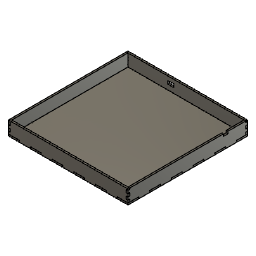
Laser cut Electronic box case v5 (Autodesk Fusion 360 design; units mm, degrees)
Autodesk Fusion 360 part; units mm, degrees
box "BoxPrimitive1" add length 215 width 215 height 3 placed x (0, 0, -1) y (-1, 0, 0) z (0, 1, 0) at (215, 0, 0) makes body 1
sketch "Sketch2" plane through (0, 0, 0) normal (0, 0, 1) x (1, 0, 0)
  line L0 (0, 3) -> (0, 0)
  line L1 (0, 0) -> (215, 0)
  line L2 (215, 0) -> (215, 3)
  line L3 (215, 3) -> (0, 3)
  line L4 (19.5455, 0) -> (39.0909, 0)
  line L5 (39.0909, 0) -> (39.0909, 3)
  line L6 (39.0909, 3) -> (19.5455, 3)
  line L7 (19.5455, 3) -> (19.5455, 0)
  dimension "d19" = 19.5455
  dimension "d20" = 3
  dimension "d21" = 19.5455
  constraint horizontal L4
  constraint vertical L5
  constraint horizontal L6
  constraint vertical L7
  constraint coincident L1 L4.start
  measures "d19" distance of L4.start L4.end
  measures "d20" distance of L4.start L6.end
  measures "d21" distance of L0.start L6.end
extrude "Extrude1" cut sketch "Sketch2" against normal blind 3 contours L1 L3 L4 L5 L6 L7 bodies 1
pattern_linear "R-Pattern1" count 5 spacing 39.0909 along (1, 0, 0) of 3 faces at (19.5455, 1, -2) (26.0606, 2, -3) (39.0909, 2, -2) on bodies 1
sketch "Sketch3" plane through (0, 0, 0) normal (-1, 0, 0) x (0, 0, 1)
  line L0 (-215, 3) -> (-215, 0)
  line L1 (-215, 0) -> (0, 0)
  line L2 (0, 0) -> (0, 3)
  line L3 (0, 3) -> (-215, 3)
  line L4 (-19.5455, 0) -> (-39.0909, 0)
  line L5 (-39.0909, 0) -> (-39.0909, 3)
  line L6 (-39.0909, 3) -> (-19.5455, 3)
  line L7 (-19.5455, 3) -> (-19.5455, 0)
  dimension "d28" = 19.5455
  dimension "d29" = 3
  dimension "d30" = 19.5455
  constraint horizontal L4
  constraint vertical L5
  constraint horizontal L6
  constraint vertical L7
  constraint coincident L1 L4.start
  measures "d28" distance of L4.start L4.end
  measures "d29" distance of L4.start L6.end
  measures "d30" distance of L2.end L6.end
extrude "Extrude2" cut sketch "Sketch3" against normal blind 3 contours L1 L3 L4 L5 L6 L7 bodies 1
pattern_linear "R-Pattern2" count 5 spacing 39.0909 along (0, 0, -1) of 3 faces at (2, 2, -39.0909) (3, 2, -32.5758) (2, 1, -19.5455) on bodies 1
sketch "Sketch4" plane through (0, 0, 0) normal (0, 0, 1) x (1, 0, 0)
  line L0 (0, 0) -> (215, 0)
  line L1 (215, 0) -> (215, 25)
  line L2 (215, 25) -> (0, 25)
  line L3 (0, 25) -> (0, 0)
  dimension "d37" = 215
  dimension "d38" = 25
  constraint horizontal L0
  constraint vertical L1
  constraint horizontal L2
  constraint vertical L3
  constraint coincident L0.start L3.end
  measures "d37" distance of L0.start L0.end
  measures "d38" distance of L0.start L2.end
extrude "Extrude3" add sketch "Sketch4" against normal blind 3 separate body makes body 2
combine "Combine1" operation cut target body 2 tool bodies 1 keep tools
sketch "Sketch6" plane through (0, 0, 0) normal (-1, 0, 0) x (0, 0, 1)
  line L0 (-3, 3) -> (0, 3)
  line L1 (0, 3) -> (0, 25)
  line L2 (0, 25) -> (-3, 25)
  line L3 (-3, 25) -> (-3, 3)
  line L4 (-3, 7.6) -> (0, 7.6)
  line L5 (0, 7.6) -> (0, 12.6)
  line L6 (0, 12.6) -> (-3, 12.6)
  line L7 (-3, 12.6) -> (-3, 7.6)
  dimension "d52" = 3
  dimension "d53" = 5
  constraint horizontal L4
  constraint vertical L5
  constraint horizontal L6
  constraint vertical L7
  constraint coincident L3 L4.start
  measures "d52" distance of L4.start L4.end
  measures "d53" distance of L4.start L6.end
extrude "Extrude7" cut sketch "Sketch6" against normal blind 3 contours L1 L3 L4 L5 L6 L7 bodies 2
pattern_linear "R-Pattern3" count 2 spacing 10 along (0, 1, 0) of 3 faces at (2, 7.6, -1) (3, 10.9333, -2) (2, 12.6, -2) on bodies 2
extrude "Extrude8" add 1 faces at (97.7273, 17.6667, -3) along direction (0, 0, 1) blind 3 from surface at -212 separate body on bodies 2 makes body 3
combine "Combine5" operation cut target body 1 tool bodies 3 keep tools
sketch "Sketch7" plane through (0, 0, 0) normal (1, 0, 0) x (0, 0, -1)
  line L0 (0, 0) -> (215, 0)
  line L1 (215, 0) -> (215, 25)
  line L2 (215, 25) -> (0, 25)
  line L3 (0, 25) -> (0, 0)
  dimension "d63" = 215
  dimension "d64" = 25
  constraint horizontal L0
  constraint vertical L1
  constraint horizontal L2
  constraint vertical L3
  constraint coincident L0.start L3.end
  measures "d63" distance of L0.start L0.end
  measures "d64" distance of L0.start L2.end
extrude "Extrude9" add sketch "Sketch7" along normal blind 3 separate body makes body 4
combine "Combine6" operation cut target body 4 tool bodies 3 1 2 keep tools
extrude "Extrude10" add 1 faces at (3, 17.6667, -97.7273) along direction (-1, 0, 0) blind 3 from surface at -212 separate body on bodies 4 makes body 5
combine "Combine7" operation cut target body 1 tool bodies 5 keep tools
combine "Combine8" operation cut target body 3 tool bodies 5 keep tools
combine "Combine9" operation cut target body 2 tool bodies 5 keep tools
sketch "Sketch8" plane through (215, 0, 0) normal (1, 0, 0) x (0, 0, -1)
  line L0 (212, 25) -> (3, 25)
  line L1 (3, 25) -> (3, 22.6)
  line L2 (3, 22.6) -> (0, 22.6)
  line L3 (0, 22.6) -> (0, 17.6)
  line L4 (0, 17.6) -> (3, 17.6)
  line L5 (3, 17.6) -> (3, 12.6)
  line L6 (3, 12.6) -> (0, 12.6)
  line L7 (0, 12.6) -> (0, 7.6)
  line L8 (0, 7.6) -> (3, 7.6)
  line L9 (3, 7.6) -> (3, 3)
  line L10 (3, 3) -> (19.5455, 3)
  line L11 (19.5455, 3) -> (19.5455, 0)
  line L12 (19.5455, 0) -> (39.0909, 0)
  line L13 (39.0909, 0) -> (39.0909, 3)
  line L14 (39.0909, 3) -> (58.6364, 3)
  line L15 (58.6364, 3) -> (58.6364, 0)
  line L16 (58.6364, 0) -> (78.1818, 0)
  line L17 (78.1818, 0) -> (78.1818, 3)
  line L18 (78.1818, 3) -> (97.7273, 3)
  line L19 (97.7273, 3) -> (97.7273, 0)
  line L20 (97.7273, 0) -> (117.2727, 0)
  line L21 (117.2727, 0) -> (117.2727, 3)
  line L22 (117.2727, 3) -> (136.8182, 3)
  line L23 (136.8182, 3) -> (136.8182, 0)
  line L24 (136.8182, 0) -> (156.3636, 0)
  line L25 (156.3636, 0) -> (156.3636, 3)
  line L26 (156.3636, 3) -> (175.9091, 3)
  line L27 (175.9091, 3) -> (175.9091, 0)
  line L28 (175.9091, 0) -> (195.4545, 0)
  line L29 (195.4545, 0) -> (195.4545, 3)
  line L30 (195.4545, 3) -> (212, 3)
  line L31 (212, 3) -> (212, 7.6)
  line L32 (212, 7.6) -> (215, 7.6)
  line L33 (215, 12.6) -> (212, 12.6)
  line L34 (212, 12.6) -> (212, 17.6)
  line L35 (212, 17.6) -> (215, 17.6)
  line L36 (215, 17.6) -> (215, 22.6)
  line L37 (215, 22.6) -> (212, 22.6)
  line L38 (212, 22.6) -> (212, 25)
  line L39 (179.8983, 25) -> (171.8983, 25)
  line L40 (171.8983, 25) -> (171.8983, 21)
  line L41 (171.8983, 21) -> (179.8983, 21)
  line L42 (179.8983, 21) -> (179.8983, 25)
  line L43 (215, 7.6) -> (215, 12.6)
  dimension "d72" = 8
  dimension "d73" = 4
  constraint horizontal L39
  constraint vertical L40
  constraint horizontal L41
  constraint vertical L42
  constraint coincident L0 L39.start
  measures "d72" distance of L39.start L39.end
  measures "d73" distance of L39.start L41.end
extrude "Extrude11" cut sketch "Sketch8" against normal blind 3 contours L0 L39 L40 L41 L42 bodies 5
sketch "Sketch9" plane through (0, 0, -215) normal (0, 0, -1) x (-1, 0, 0)
  line L0 (-212, 7.6) -> (-215, 7.6)
  line L1 (-215, 7.6) -> (-215, 3)
  line L2 (-215, 3) -> (-195.4545, 3)
  line L3 (-195.4545, 3) -> (-195.4545, 0)
  line L4 (-195.4545, 0) -> (-175.9091, 0)
  line L5 (-175.9091, 0) -> (-175.9091, 3)
  line L6 (-175.9091, 3) -> (-156.3636, 3)
  line L7 (-156.3636, 3) -> (-156.3636, 0)
  line L8 (-156.3636, 0) -> (-136.8182, 0)
  line L9 (-136.8182, 0) -> (-136.8182, 3)
  line L10 (-136.8182, 3) -> (-117.2727, 3)
  line L11 (-117.2727, 3) -> (-117.2727, 0)
  line L12 (-117.2727, 0) -> (-97.7273, 0)
  line L13 (-97.7273, 0) -> (-97.7273, 3)
  line L14 (-97.7273, 3) -> (-78.1818, 3)
  line L15 (-78.1818, 3) -> (-78.1818, 0)
  line L16 (-78.1818, 0) -> (-58.6364, 0)
  line L17 (-58.6364, 0) -> (-58.6364, 3)
  line L18 (-58.6364, 3) -> (-39.0909, 3)
  line L19 (-39.0909, 3) -> (-39.0909, 0)
  line L20 (-39.0909, 0) -> (-19.5455, 0)
  line L21 (-19.5455, 0) -> (-19.5455, 3)
  line L22 (-19.5455, 3) -> (0, 3)
  line L23 (0, 3) -> (0, 7.6)
  line L24 (0, 7.6) -> (-3, 7.6)
  line L25 (-3, 7.6) -> (-3, 12.6)
  line L26 (-3, 12.6) -> (0, 12.6)
  line L27 (0, 12.6) -> (0, 17.6)
  line L28 (0, 17.6) -> (-3, 17.6)
  line L29 (-3, 17.6) -> (-3, 22.6)
  line L30 (-3, 22.6) -> (0, 22.6)
  line L31 (0, 22.6) -> (0, 25)
  line L32 (0, 25) -> (-215, 25)
  line L33 (-215, 22.6) -> (-212, 22.6)
  line L34 (-212, 22.6) -> (-212, 17.6)
  line L35 (-212, 17.6) -> (-215, 17.6)
  line L36 (-215, 12.6) -> (-212, 12.6)
  line L37 (-74.7061, 17.8863) -> (-85.2061, 17.8863)
  line L38 (-85.2061, 17.8863) -> (-85.2061, 12.1863)
  line L39 (-85.2061, 12.1863) -> (-74.7061, 12.1863)
  line L40 (-74.7061, 12.1863) -> (-74.7061, 17.8863)
  line L41 (-74.7061, 17.8863) -> (-85.2061, 12.1863) construction
  line L42 (-85.2061, 17.8863) -> (-74.7061, 12.1863) construction
  line L43 (-215, 25) -> (-215, 22.6)
  line L44 (-215, 17.6) -> (-215, 12.6)
  line L45 (-212, 12.6) -> (-212, 7.6)
  point P0 (-79.9561, 15.0363)
  dimension "d78" = 10.5
  dimension "d79" = 5.7
  constraint horizontal L37
  constraint perpendicular L37 L38
  constraint parallel L37 L39
  constraint parallel L38 L40
  constraint coincident L41 P0
  constraint coincident L42 P0
  measures "d78" distance of L38.end L39.end
  measures "d79" distance of L37.end L38.end
extrude "Extrude12" cut sketch "Sketch9" against normal blind 3 contours L37 L38 L39 L40 bodies 3
sketch "Base DXF" plane through (0, 3, 0) normal (0, 1, 0) x (-1, 0, 0)
  line L0 (-215, 0) -> (-215, -19.5455)
  line L1 (-215, -19.5455) -> (-212, -19.5455)
  line L2 (-212, -19.5455) -> (-212, -39.0909)
  line L3 (-212, -39.0909) -> (-215, -39.0909)
  line L4 (-215, -39.0909) -> (-215, -58.6364)
  line L5 (-215, -58.6364) -> (-212, -58.6364)
  line L6 (-212, -58.6364) -> (-212, -78.1818)
  line L7 (-212, -78.1818) -> (-215, -78.1818)
  line L8 (-215, -78.1818) -> (-215, -97.7273)
  line L9 (-215, -97.7273) -> (-212, -97.7273)
  line L10 (-212, -97.7273) -> (-212, -117.2727)
  line L11 (-212, -117.2727) -> (-215, -117.2727)
  line L12 (-215, -117.2727) -> (-215, -136.8182)
  line L13 (-215, -136.8182) -> (-212, -136.8182)
  line L14 (-212, -136.8182) -> (-212, -156.3636)
  line L15 (-212, -156.3636) -> (-215, -156.3636)
  line L16 (-215, -156.3636) -> (-215, -175.9091)
  line L17 (-215, -175.9091) -> (-212, -175.9091)
  line L18 (-212, -175.9091) -> (-212, -195.4545)
  line L19 (-212, -195.4545) -> (-215, -195.4545)
  line L20 (-215, -195.4545) -> (-215, -215)
  line L21 (-215, -215) -> (-195.4545, -215)
  line L22 (-195.4545, -215) -> (-195.4545, -212)
  line L23 (-195.4545, -212) -> (-175.9091, -212)
  line L24 (-175.9091, -212) -> (-175.9091, -215)
  line L25 (-175.9091, -215) -> (-156.3636, -215)
  line L26 (-156.3636, -215) -> (-156.3636, -212)
  line L27 (-156.3636, -212) -> (-136.8182, -212)
  line L28 (-136.8182, -212) -> (-136.8182, -215)
  line L29 (-136.8182, -215) -> (-117.2727, -215)
  line L30 (-117.2727, -215) -> (-117.2727, -212)
  line L31 (-117.2727, -212) -> (-97.7273, -212)
  line L32 (-97.7273, -212) -> (-97.7273, -215)
  line L33 (-97.7273, -215) -> (-78.1818, -215)
  line L34 (-78.1818, -215) -> (-78.1818, -212)
  line L35 (-78.1818, -212) -> (-58.6364, -212)
  line L36 (-58.6364, -212) -> (-58.6364, -215)
  line L37 (-58.6364, -215) -> (-39.0909, -215)
  line L38 (-39.0909, -215) -> (-39.0909, -212)
  line L39 (-39.0909, -212) -> (-19.5455, -212)
  line L40 (-19.5455, -212) -> (-19.5455, -215)
  line L41 (-19.5455, -215) -> (0, -215)
  line L42 (0, -215) -> (0, -195.4545)
  line L43 (0, -195.4545) -> (-3, -195.4545)
  line L44 (-3, -195.4545) -> (-3, -175.9091)
  line L45 (-3, -175.9091) -> (0, -175.9091)
  line L46 (0, -175.9091) -> (0, -156.3636)
  line L47 (0, -156.3636) -> (-3, -156.3636)
  line L48 (-3, -156.3636) -> (-3, -136.8182)
  line L49 (-3, -136.8182) -> (0, -136.8182)
  line L50 (0, -136.8182) -> (0, -117.2727)
  line L51 (0, -117.2727) -> (-3, -117.2727)
  line L52 (-3, -117.2727) -> (-3, -97.7273)
  line L53 (-3, -97.7273) -> (0, -97.7273)
  line L54 (0, -97.7273) -> (0, -78.1818)
  line L55 (0, -78.1818) -> (-3, -78.1818)
  line L56 (-3, -78.1818) -> (-3, -58.6364)
  line L57 (-3, -58.6364) -> (0, -58.6364)
  line L58 (0, -58.6364) -> (0, -39.0909)
  line L59 (0, -39.0909) -> (-3, -39.0909)
  line L60 (-3, -39.0909) -> (-3, -19.5455)
  line L61 (-3, -19.5455) -> (0, -19.5455)
  line L62 (0, -19.5455) -> (0, 0)
  line L63 (0, 0) -> (-19.5455, 0)
  line L64 (-19.5455, 0) -> (-19.5455, -3)
  line L65 (-19.5455, -3) -> (-39.0909, -3)
  line L66 (-39.0909, -3) -> (-39.0909, 0)
  line L67 (-39.0909, 0) -> (-58.6364, 0)
  line L68 (-58.6364, 0) -> (-58.6364, -3)
  line L69 (-58.6364, -3) -> (-78.1818, -3)
  line L70 (-78.1818, -3) -> (-78.1818, 0)
  line L71 (-78.1818, 0) -> (-97.7273, 0)
  line L72 (-97.7273, 0) -> (-97.7273, -3)
  line L73 (-97.7273, -3) -> (-117.2727, -3)
  line L74 (-117.2727, -3) -> (-117.2727, 0)
  line L75 (-117.2727, 0) -> (-136.8182, 0)
  line L76 (-136.8182, 0) -> (-136.8182, -3)
  line L77 (-136.8182, -3) -> (-156.3636, -3)
  line L78 (-156.3636, -3) -> (-156.3636, 0)
  line L79 (-156.3636, 0) -> (-175.9091, 0)
  line L80 (-175.9091, 0) -> (-175.9091, -3)
  line L81 (-175.9091, -3) -> (-195.4545, -3)
  line L82 (-195.4545, -3) -> (-195.4545, 0)
  line L83 (-195.4545, 0) -> (-215, 0)
sketch "Front DXF" plane through (0, 0, 0) normal (0, 0, 1) x (1, 0, 0)
  line L0 (212, 22.6) -> (215, 22.6)
  line L1 (215, 22.6) -> (215, 25)
  line L2 (215, 25) -> (0, 25)
  line L3 (0, 25) -> (0, 22.6)
  line L4 (0, 22.6) -> (3, 22.6)
  line L5 (3, 22.6) -> (3, 17.6)
  line L6 (3, 17.6) -> (0, 17.6)
  line L7 (0, 17.6) -> (0, 12.6)
  line L8 (0, 12.6) -> (3, 12.6)
  line L9 (3, 12.6) -> (3, 7.6)
  line L10 (3, 7.6) -> (0, 7.6)
  line L11 (0, 7.6) -> (0, 3)
  line L12 (0, 3) -> (19.5455, 3)
  line L13 (19.5455, 3) -> (19.5455, 0)
  line L14 (19.5455, 0) -> (39.0909, 0)
  line L15 (39.0909, 0) -> (39.0909, 3)
  line L16 (39.0909, 3) -> (58.6364, 3)
  line L17 (58.6364, 3) -> (58.6364, 0)
  line L18 (58.6364, 0) -> (78.1818, 0)
  line L19 (78.1818, 0) -> (78.1818, 3)
  line L20 (78.1818, 3) -> (97.7273, 3)
  line L21 (97.7273, 3) -> (97.7273, 0)
  line L22 (97.7273, 0) -> (117.2727, 0)
  line L23 (117.2727, 0) -> (117.2727, 3)
  line L24 (117.2727, 3) -> (136.8182, 3)
  line L25 (136.8182, 3) -> (136.8182, 0)
  line L26 (136.8182, 0) -> (156.3636, 0)
  line L27 (156.3636, 0) -> (156.3636, 3)
  line L28 (156.3636, 3) -> (175.9091, 3)
  line L29 (175.9091, 3) -> (175.9091, 0)
  line L30 (175.9091, 0) -> (195.4545, 0)
  line L31 (195.4545, 0) -> (195.4545, 3)
  line L32 (195.4545, 3) -> (215, 3)
  line L33 (215, 3) -> (215, 7.6)
  line L34 (215, 7.6) -> (212, 7.6)
  line L35 (212, 7.6) -> (212, 12.6)
  line L36 (212, 12.6) -> (215, 12.6)
  line L37 (215, 12.6) -> (215, 17.6)
  line L38 (215, 17.6) -> (212, 17.6)
  line L39 (212, 17.6) -> (212, 22.6)
sketch "Back DXF" plane through (0, 0, -215) normal (0, 0, -1) x (-1, 0, 0)
  line L0 (-85.2061, 17.8863) -> (-74.7061, 17.8863)
  line L1 (-74.7061, 17.8863) -> (-74.7061, 12.1863)
  line L2 (-74.7061, 12.1863) -> (-85.2061, 12.1863)
  line L3 (-85.2061, 12.1863) -> (-85.2061, 17.8863)
  line L4 (-212, 7.6) -> (-215, 7.6)
  line L5 (-215, 7.6) -> (-215, 3)
  line L6 (-215, 3) -> (-195.4545, 3)
  line L7 (-195.4545, 3) -> (-195.4545, 0)
  line L8 (-195.4545, 0) -> (-175.9091, 0)
  line L9 (-175.9091, 0) -> (-175.9091, 3)
  line L10 (-175.9091, 3) -> (-156.3636, 3)
  line L11 (-156.3636, 3) -> (-156.3636, 0)
  line L12 (-156.3636, 0) -> (-136.8182, 0)
  line L13 (-136.8182, 0) -> (-136.8182, 3)
  line L14 (-136.8182, 3) -> (-117.2727, 3)
  line L15 (-117.2727, 3) -> (-117.2727, 0)
  line L16 (-117.2727, 0) -> (-97.7273, 0)
  line L17 (-97.7273, 0) -> (-97.7273, 3)
  line L18 (-97.7273, 3) -> (-78.1818, 3)
  line L19 (-78.1818, 3) -> (-78.1818, 0)
  line L20 (-78.1818, 0) -> (-58.6364, 0)
  line L21 (-58.6364, 0) -> (-58.6364, 3)
  line L22 (-58.6364, 3) -> (-39.0909, 3)
  line L23 (-39.0909, 3) -> (-39.0909, 0)
  line L24 (-39.0909, 0) -> (-19.5455, 0)
  line L25 (-19.5455, 0) -> (-19.5455, 3)
  line L26 (-19.5455, 3) -> (0, 3)
  line L27 (0, 3) -> (0, 7.6)
  line L28 (0, 7.6) -> (-3, 7.6)
  line L29 (-3, 7.6) -> (-3, 12.6)
  line L30 (-3, 12.6) -> (0, 12.6)
  line L31 (0, 12.6) -> (0, 17.6)
  line L32 (0, 17.6) -> (-3, 17.6)
  line L33 (-3, 17.6) -> (-3, 22.6)
  line L34 (-3, 22.6) -> (0, 22.6)
  line L35 (0, 22.6) -> (0, 25)
  line L36 (0, 25) -> (-215, 25)
  line L37 (-215, 25) -> (-215, 22.6)
  line L38 (-215, 22.6) -> (-212, 22.6)
  line L39 (-212, 22.6) -> (-212, 17.6)
  line L40 (-212, 17.6) -> (-215, 17.6)
  line L41 (-215, 17.6) -> (-215, 12.6)
  line L42 (-215, 12.6) -> (-212, 12.6)
  line L43 (-212, 12.6) -> (-212, 7.6)
sketch "Right DXF" plane through (215, 0, 0) normal (1, 0, 0) x (0, 0, -1)
  line L0 (171.8983, 21) -> (171.8983, 25)
  line L1 (171.8983, 25) -> (3, 25)
  line L2 (3, 25) -> (3, 22.6)
  line L3 (3, 22.6) -> (0, 22.6)
  line L4 (0, 22.6) -> (0, 17.6)
  line L5 (0, 17.6) -> (3, 17.6)
  line L6 (3, 17.6) -> (3, 12.6)
  line L7 (3, 12.6) -> (0, 12.6)
  line L8 (0, 12.6) -> (0, 7.6)
  line L9 (0, 7.6) -> (3, 7.6)
  line L10 (3, 7.6) -> (3, 3)
  line L11 (3, 3) -> (19.5455, 3)
  line L12 (19.5455, 3) -> (19.5455, 0)
  line L13 (19.5455, 0) -> (39.0909, 0)
  line L14 (39.0909, 0) -> (39.0909, 3)
  line L15 (39.0909, 3) -> (58.6364, 3)
  line L16 (58.6364, 3) -> (58.6364, 0)
  line L17 (58.6364, 0) -> (78.1818, 0)
  line L18 (78.1818, 0) -> (78.1818, 3)
  line L19 (78.1818, 3) -> (97.7273, 3)
  line L20 (97.7273, 3) -> (97.7273, 0)
  line L21 (97.7273, 0) -> (117.2727, 0)
  line L22 (117.2727, 0) -> (117.2727, 3)
  line L23 (117.2727, 3) -> (136.8182, 3)
  line L24 (136.8182, 3) -> (136.8182, 0)
  line L25 (136.8182, 0) -> (156.3636, 0)
  line L26 (156.3636, 0) -> (156.3636, 3)
  line L27 (156.3636, 3) -> (175.9091, 3)
  line L28 (175.9091, 3) -> (175.9091, 0)
  line L29 (175.9091, 0) -> (195.4545, 0)
  line L30 (195.4545, 0) -> (195.4545, 3)
  line L31 (195.4545, 3) -> (212, 3)
  line L32 (212, 3) -> (212, 7.6)
  line L33 (212, 7.6) -> (215, 7.6)
  line L34 (215, 7.6) -> (215, 12.6)
  line L35 (215, 12.6) -> (212, 12.6)
  line L36 (212, 12.6) -> (212, 17.6)
  line L37 (212, 17.6) -> (215, 17.6)
  line L38 (215, 17.6) -> (215, 22.6)
  line L39 (215, 22.6) -> (212, 22.6)
  line L40 (212, 22.6) -> (212, 25)
  line L41 (212, 25) -> (179.8983, 25)
  line L42 (179.8983, 25) -> (179.8983, 21)
  line L43 (179.8983, 21) -> (171.8983, 21)
sketch "Left DXF" plane through (0, 0, 0) normal (-1, 0, 0) x (0, 0, 1)
  line L0 (-3, 22.6) -> (-3, 25)
  line L1 (-3, 25) -> (-212, 25)
  line L2 (-212, 25) -> (-212, 22.6)
  line L3 (-212, 22.6) -> (-215, 22.6)
  line L4 (-215, 22.6) -> (-215, 17.6)
  line L5 (-215, 17.6) -> (-212, 17.6)
  line L6 (-212, 17.6) -> (-212, 12.6)
  line L7 (-212, 12.6) -> (-215, 12.6)
  line L8 (-215, 12.6) -> (-215, 7.6)
  line L9 (-215, 7.6) -> (-212, 7.6)
  line L10 (-212, 7.6) -> (-212, 3)
  line L11 (-212, 3) -> (-195.4545, 3)
  line L12 (-195.4545, 3) -> (-195.4545, 0)
  line L13 (-195.4545, 0) -> (-175.9091, 0)
  line L14 (-175.9091, 0) -> (-175.9091, 3)
  line L15 (-175.9091, 3) -> (-156.3636, 3)
  line L16 (-156.3636, 3) -> (-156.3636, 0)
  line L17 (-156.3636, 0) -> (-136.8182, 0)
  line L18 (-136.8182, 0) -> (-136.8182, 3)
  line L19 (-136.8182, 3) -> (-117.2727, 3)
  line L20 (-117.2727, 3) -> (-117.2727, 0)
  line L21 (-117.2727, 0) -> (-97.7273, 0)
  line L22 (-97.7273, 0) -> (-97.7273, 3)
  line L23 (-97.7273, 3) -> (-78.1818, 3)
  line L24 (-78.1818, 3) -> (-78.1818, 0)
  line L25 (-78.1818, 0) -> (-58.6364, 0)
  line L26 (-58.6364, 0) -> (-58.6364, 3)
  line L27 (-58.6364, 3) -> (-39.0909, 3)
  line L28 (-39.0909, 3) -> (-39.0909, 0)
  line L29 (-39.0909, 0) -> (-19.5455, 0)
  line L30 (-19.5455, 0) -> (-19.5455, 3)
  line L31 (-19.5455, 3) -> (-3, 3)
  line L32 (-3, 3) -> (-3, 7.6)
  line L33 (-3, 7.6) -> (0, 7.6)
  line L34 (0, 7.6) -> (0, 12.6)
  line L35 (0, 12.6) -> (-3, 12.6)
  line L36 (-3, 12.6) -> (-3, 17.6)
  line L37 (-3, 17.6) -> (0, 17.6)
  line L38 (0, 17.6) -> (0, 22.6)
  line L39 (0, 22.6) -> (-3, 22.6)
equation "Length = 215 mm"
equation "Width = 215 mm"
equation "Height = 25 mm"
equation "Thickness = 3 mm"
equation "LSTab = 5"
equation "WSTab = 5"
equation "HSTab = 2"
equation "LTabForm = Length / ( ( LSTab * 2 ) + 1 )"
equation "WTabForm = Width / ( ( WSTab * 2 ) + 1 )"
equation "HTabForm = Height / ( ( HSTab * 2 ) + 1 )"
equation "LPattForm = ( Length - ( LTabForm * 3 ) )"
equation "WPattForm = ( Width - ( WTabForm * 3 ) )"
equation "HPattForm = ( Height - ( HTabForm * 3 ) )"
equation "d14 = Width"
equation "d15 = Length"
equation "d16 = Thickness"
equation "d19 = LTabForm"
equation "d20 = Thickness"
equation "d21 = LTabForm"
equation "d22 = -Thickness"
equation "d24 = LSTab"
equation "d26 = -LPattForm"
equation "d28 = WTabForm"
equation "d29 = Thickness"
equation "d30 = WTabForm"
equation "d31 = -Thickness"
equation "d33 = WSTab"
equation "d35 = WPattForm"
equation "d37 = Length"
equation "d38 = Height"
equation "d39 = -Thickness"
equation "d52 = Thickness"
equation "d53 = HTabForm"
equation "d54 = -Thickness"
equation "d56 = HSTab"
equation "d58 = -HPattForm"
equation "d61 = -Thickness"
equation "d63 = Width"
equation "d64 = Height"
equation "d65 = Thickness"
equation "d68 = -Thickness"
equation "LServoWireHole = 8 mm"
equation "HServoWireHole = 4 mm"
equation "d72 = LServoWireHole"
equation "d73 = HServoWireHole"
equation "d74 = -Thickness"
equation "HSlideSWHole = 5.7 mm"
equation "LSlideSWHole = 10.5 mm"
equation "d78 = LSlideSWHole"
equation "d79 = HSlideSWHole"
equation "d80 = -Thickness"
named bodies: "Base", "Front", "Back", "Left", "Right"
